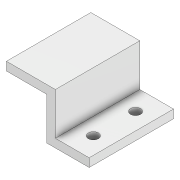
# Autodesk Inventor part: Carcasa para Reed Switch
Saved by Autodesk Inventor 2020 (Build 240168000, 168)
## iProperties
Created: 2020-10-01
Part Number: Carcasa para Reed Switch
Material: ABS Plastic
Document SubType Name: Modeling
Designer: Hernan
Density: 1.06 g/cm^3
Appearance: Smooth - White
Author: Hernan
Autodesk Inventor part; units mm, degrees
ref_plane "YZ Plane" through (0, 0, 0) normal (1, 0, 0) x (0, 1, 0)
ref_plane "XZ Plane" through (0, 0, 0) normal (0, 1, 0) x (-1, 0, 0)
ref_plane "XY Plane" through (0, 0, 0) normal (0, 0, 1) x (1, 0, 0)
sketch "Sketch1" plane through (0, 0, 0) normal (0, 0, 1) x (1, 0, 0)
  line L0 (-9.0446, 8.8114) -> (-9.0446, -3.6886)
  line L1 (-11.5446, 6.3114) -> (-11.5446, -6.1886)
  line L2 (-9.0446, -3.6886) -> (0.9554, -3.6886)
  line L3 (0.9554, -3.6886) -> (0.9554, -6.1886)
  line L4 (0.9554, -6.1886) -> (-11.5446, -6.1886)
  line L5 (-23.5446, 8.8114) -> (-23.5446, 6.3114)
  line L6 (-23.5446, 6.3114) -> (-11.5446, 6.3114)
  line L7 (-23.5446, 8.8114) -> (-9.0446, 8.8114)
  point P0 (0, 0)
  dimension "d22" = 2.5
  dimension "d39" = 10
  dimension "d48" = 24.5
  constraints: 16 end point, 2 horizontal, 2 perpendicular, 1 parallel, 1 vertical
  measures "d22" distance between parallel lines of L1 L0
  measures "d39" distance of L0.end L2.end
  measures "d48" distance between parallel lines of L3 L5
extrude "Extrusion1" add sketch "Sketch1" against normal blind 25
sketch "Sketch5" plane through (-9.0446, -3.6886, 0) normal (0, 1, 0) x (1, 0, 0)
  line L0 (10, 0) -> (10, 25) projected
  line L1 (10, 12.5) -> (0, 12.5)
  line L2 (0, 0) -> (0, 25) projected
  line L3 (0, 25) -> (10, 25) projected
  line L4 (5, 25) -> (5, 0)
  line L5 (-2.5, 0) -> (10, 0) projected
  line L6 (0, 0) -> (0, 25) projected
  line L7 (0, 6.25) -> (10, 6.25)
  line L8 (10, 0) -> (10, 25) projected
  line L9 (0, 18.75) -> (10, 18.75)
  circle A0 centre (5, 18.75) radius 1.5
  circle A1 centre (5, 6.25) radius 1.5
  point P0 (9.0446, 0)
  dimension "d49" = 6.25
  dimension "d50" = 6.25
  dimension "d51" = 3
  dimension "d52" = 3
  constraints: 8 end point, 5 midpoint, 5 point on line, 3 perpendicular, 2 centre point
  measures "d49" distance between parallel lines of L5 L7
  measures "d50" distance between parallel lines of L3 L9
  measures "d51" diameter of A0
  measures "d52" diameter of A1
extrude "Extrusion5" cut sketch "Sketch5" against normal blind 4 contours A1 L4 L7 | L7 L4 A1 | A1 L7 L4 | L7 A1 L4 | A0 L4 L9 | L9 L4 A0 | A0 L9 L4 | L9 A0 L4
body "Solid1"
